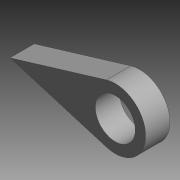
# Autodesk Inventor part: Body
Saved by Autodesk Inventor 2014 SP1 (Build 180222100, 222)
## iProperties
Created: 2013-12-25
Part Number: Body
Material: Generic
Document SubType Name: Modeling
Designer: tom
Density: 1 g/cm^3
Appearance: Default
Author: tom
Autodesk Inventor part; units mm, degrees
ref_plane "YZ Plane" through (0, 0, 0) normal (1, 0, 0) x (0, 1, 0)
ref_plane "XZ Plane" through (0, 0, 0) normal (0, 1, 0) x (-1, 0, 0)
ref_plane "XY Plane" through (0, 0, 0) normal (0, 0, 1) x (1, 0, 0)
sketch "Sketch1" plane through (0, 0, 0) normal (0, 0, 1) x (1, 0, 0)
  arc A0 (-1.539, -5.0978) -> (-1.539, 5.0978) centre (0, 0) ccw
  line L0 (-18.425, 0) -> (-1.539, -5.0978)
  line L1 (-18.425, 0) -> (-1.539, 5.0978)
  circle A1 centre (0, 0) radius 3.5
  dimension "d0" = 10.65
  dimension "d2" = 7
  constraints: 4 end point, 2 centre point, 2 coincident, 2 point on circle, 2 tangent
  measures "d0" diameter of A0
  measures "d2" diameter of A1
extrude "Extrusion1" add sketch "Sketch1" along normal mid plane 4.25
sketch "Sketch2" plane through (0, 0, 0) normal (0, 0, 1) x (1, 0, 0)
  circle A0 centre (0, 0) radius 3.5
  dimension "d5" = 7
  constraints: 1 centre point, 1 coincident
  measures "d5" diameter of A0
extrude "Extrusion2" add sketch "Sketch2" along normal mid plane 3.75
sketch "Sketch3" plane through (0, 0, 0) normal (0, 0, 1) x (1, 0, 0)
  circle A0 centre (0, 0) radius 3.175
  line L0 (0, 0) -> (0, -3.7497)
  line L1 (0, -3.7497) -> (0, 0)
  line L2 (0, -0.8126) -> (0, 3.6567)
  line L3 (3.175, 0) -> (-3.175, 0)
  dimension "d8" = 6.35
  constraints: 8 end point, 2 point on circle, 2 point on line, 1 centre point, 1 coincident, 1 collinear, 1 perpendicular, 1 vertical
  measures "d8" diameter of A0
revolve "Revolution1" cut sketch "Sketch3" angle 360 about axis through (3.175, 0, 0) along (-1, 0, 0) contours A0 L0 L3 | A0 L3 L0
body "Solid1"
